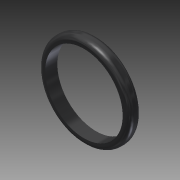
# Autodesk Inventor part: Wheel_Tire
Saved by Autodesk Inventor 2013 (Build 170138000, 138)
## iProperties
Created: 2015-07-06
Part Number: Wheel_Tire
Material: Rubber, Silicone
Document SubType Name: Modeling
Designer: Kyle
Density: 1.25 g/cm^3
Mass: 6.84439 g
Surface Area: 38.3511 cm^2
Volume: 5.47551 cm^3
Author: Kyle
Autodesk Inventor part; units mm, degrees
ref_plane "YZ Plane" through (0, 0, 0) normal (1, 0, 0) x (0, 1, 0)
ref_plane "XZ Plane" through (0, 0, 0) normal (0, 1, 0) x (-1, 0, 0)
ref_plane "XY Plane" through (0, 0, 0) normal (0, 0, 1) x (1, 0, 0)
sketch "Sketch1" plane through (0, 0, 0) normal (0, 0, 1) x (1, 0, 0)
  circle A0 centre (0, 0) radius 29.9974
  circle A1 centre (0, 0) radius 25.5016
  dimension "d0" = 59.9948
  dimension "d2" = 51.0032
  constraints: 2 centre point, 2 coincident
  measures "d0" diameter of A0
  measures "d2" diameter of A1
extrude "Extrusion1" add sketch "Sketch1" along normal blind 8.001
fillet "Fillet1" radius 3.175 2 edges at (-29.9974, 0, 8.001) (-29.9974, 0, 0)
body "Solid1"
